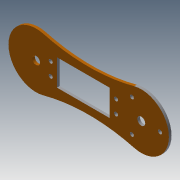
# Autodesk Inventor part: dibond_strana(b)
Saved by Autodesk Inventor 2013 (Build 170138000, 138)
## iProperties
Created: 2013-05-11
Part Number: dibond_strana(b)
Material: Generic
Document SubType Name: Modeling
Designer: idle-rug
Density: 1 g/cm^3
Author: idle-rug
Autodesk Inventor part; units mm, degrees
ref_plane "YZ Plane" through (0, 0, 0) normal (1, 0, 0) x (0, 1, 0)
ref_plane "XZ Plane" through (0, 0, 0) normal (0, 1, 0) x (-1, 0, 0)
ref_plane "XY Plane" through (0, 0, 0) normal (0, 0, 1) x (1, 0, 0)
sketch "Sketch1" plane through (0, 0, 0) normal (0, 1, 0) x (-1, 0, 0)
  line L0 (-50.5, -21) -> (-38.580998, -21)
  line L1 (-50.5, -21) -> (-38.580998, -21)
  line L2 (-50.5, 21) -> (-38.580998, 21)
  arc A0 (-50.5, 21) -> (-50.5, -21) centre (-50.5, 0) ccw
  circle A1 centre (40, 0) radius 3
  line L3 (-71.5, 0) -> (-61.5, 0)
  line L4 (-50.5, 21) -> (-37.146287, 21)
  arc A2 (-37.146287, 21) -> (34.589084, 20.290934) centre (0, 150) ccw
  line L5 (-50.5, -21) -> (-37.146287, -21)
  arc A3 (34.589084, -20.290934) -> (-37.146287, -21) centre (0, -150) ccw
  circle A4 centre (-61.5, 0) radius 2
  line L6 (40, 0) -> (20, 0)
  circle A5 centre (20, 0) radius 2
  arc A6 (37.224562, -20.815786) -> (37.224562, 20.815786) centre (40, 0) ccw
  arc A7 (34.589084, -20.290934) -> (34.589084, 20.290934) centre (40, 0) ccw
  point P0 (0, 0)
  point P1 (0, 0)
  dimension "d1" = 6
  dimension "d3" = 10
  dimension "d5" = 4
  dimension "d7" = 4
  constraints: 14 end point, 11 point on circle, 8 centre point, 5 tangent, 2 coincident, 1 point on line
  measures "d1" diameter of A1
  measures "d3" distance of L3.start L3.end
  measures "d5" diameter of A4
  measures "d7" diameter of A5
extrude "Extrusion1" add sketch "Sketch1" along normal blind 2
sketch "Sketch2" plane through (0, 2, 0) normal (0, 1, 0) x (1, 0, 0)
  circle A0 centre (-54.25, 0) radius 1.5
  circle A1 centre (-32.875, 12.340862) radius 1.5
  circle A2 centre (-32.875, -12.340862) radius 1.5
  point P0 (0, 0)
  dimension "d11" = 3
  dimension "d14" = 3
  dimension "d15" = 3
  constraints: 3 centre point
  measures "d11" diameter of A0
  measures "d14" diameter of A1
  measures "d15" diameter of A2
extrude "Extrusion2" cut sketch "Sketch2" against normal blind 2
sketch "Sketch3" plane through (0, 2, 0) normal (0, 1, 0) x (1, 0, 0)
  line L0 (37.146287, -21) -> (50.5, -21)
  arc A0 (50.5, -21) -> (50.5, 21) centre (50.5, 0) ccw
  line L1 (50.5, 0) -> (40, 0)
  circle A1 centre (40, 0) radius 3
  point P0 (0, 0)
  dimension "d18" = 10.5
  dimension "d19" = 6
  constraints: 2 end point, 1 centre point, 1 coincident, 1 parallel
  measures "d18" distance of L1.start L1.end
  measures "d19" diameter of A1
extrude "Extrusion3" cut sketch "Sketch3" against normal blind 2
sketch "Sketch4" plane through (0, 0, 0) normal (0, -1, 0) x (1, 0, 0)
  circle A0 centre (40, 0) radius 3
  line L0 (40, 0) -> (54.25, 0) construction
  line L1 (40, 0) -> (54.25, 0) construction
  line L2 (40, 0) -> (54.25, 0) construction
  line L3 (40, 0) -> (54.25, 0) construction
  circle A1 centre (47.125, 12.340862) radius 1.5
  circle A2 centre (25.75, 0) radius 1.5
  circle A3 centre (47.125, -12.340862) radius 1.5
  point P0 (0, 0)
  dimension "d33" = 3
  dimension "d34" = 3
  dimension "d35" = 3
  constraints: 8 end point, 4 horizontal, 3 centre point, 1 coincident
  measures "d33" diameter of A1
  measures "d34" diameter of A2
  measures "d35" diameter of A3
extrude "Extrusion4" cut sketch "Sketch4" against normal blind 2 contours A1 | A2 | A3
sketch "Sketch5" plane through (0, 0, 0) normal (0, -1, 0) x (1, 0, 0)
  line L0 (50.5, -21) -> (37.146287, -21)
  arc A0 (50.5, -21) -> (50.5, 21) centre (50.5, 0) ccw
  line L1 (37.146287, 21) -> (50.5, 21)
  arc A1 (-34.589084, 20.290934) -> (37.146287, 21) centre (0, 150) ccw
  arc A2 (-34.589084, 20.290934) -> (-34.589084, -20.290934) centre (-40, 0) ccw
  arc A3 (37.146287, -21) -> (-34.589084, -20.290934) centre (0, -150) ccw
  line L2 (74.65, 0) -> (104.15, 0)
  line L3 (74.65, 0) -> (63.95, 0)
  line L4 (37.146287, 21) -> (104.15, 21)
  line L5 (104.15, 21) -> (37.146287, 21)
  line L6 (37.146287, -21) -> (104.15, -21)
  line L7 (63.95, 0) -> (104.15, 0)
  line L8 (104.15, 10) -> (63.95, 10)
  line L9 (63.95, 10) -> (63.95, -10)
  line L10 (63.95, -10) -> (104.15, -10)
  line L11 (104.15, -10) -> (104.15, 10)
  line L12 (104.15, 10) -> (63.95, -10) construction
  line L13 (63.95, 10) -> (104.15, -10) construction
  line L14 (104.15, -4.95) -> (104.15, -10)
  line L15 (104.15, 4.95) -> (104.15, 10)
  arc A4 (104.15, -21) -> (104.15, 21) centre (104.15, 0) ccw
  circle A5 centre (108.9, 4.95) radius 1.5
  circle A6 centre (108.9, -4.95) radius 1.5
  circle A7 centre (59.2, 4.95) radius 1.5
  circle A8 centre (59.2, -4.95) radius 1.5
  point P0 (0, 0)
  point P1 (84.05, 0)
  dimension "d46" = 29.5
  dimension "d48" = 10.7
  dimension "d49" = 40.2
  dimension "d57" = 3
  dimension "d58" = 3
  constraints: 28 end point, 5 centre point, 5 parallel, 3 midpoint, 2 collinear, 2 horizontal, 2 point on circle, 2 tangent, 1 perpendicular
  measures "d46" distance of L2.start L2.end
  measures "d48" distance of L2.start L3.end
  measures "d49" distance of L10.end L9.end
  measures "d57" diameter of A5
  measures "d58" diameter of A6
extrude "Extrusion5" add sketch "Sketch5" against normal blind 2 contours A0 L10 L11 L8 L4 A4 L6
sketch "Sketch6" plane through (0, 0, 0) normal (0, -1, 0) x (1, 0, 0)
  arc A0 (68.966185, -10) -> (68.966185, 10) centre (50.5, 0) ccw
  line L0 (68.966185, 10) -> (104.15, 10)
  line L1 (104.15, 10) -> (104.15, -10)
  line L2 (104.15, -10) -> (68.966185, -10)
  line L3 (104.15, 10) -> (63.95, 10)
  line L4 (63.95, 10) -> (63.95, -10)
  line L5 (63.95, -10) -> (104.15, -10)
  line L6 (104.15, -10) -> (104.15, 10)
  point P0 (0, 0)
  dimension "d65" = 40.2
  dimension "d66" = 20
  constraints: 8 end point, 1 collinear, 1 perpendicular, 1 point on line
  measures "d65" distance of L0.end L3.end
  measures "d66" distance of L3.end L4.end
extrude "Extrusion6" cut sketch "Sketch6" against normal blind 2 contours L5 L4 L3 A0
sketch "Sketch7" plane through (0, 0, 0) normal (0, -1, 0) x (1, 0, 0)
  circle A0 centre (61.5, 0) radius 2 projected
  point P0 (0, 0)
extrude "Extrusion7" add sketch "Sketch7" against normal blind 2
sketch "Sketch8" plane through (0, 0, 0) normal (0, -1, 0) x (1, 0, 0)
  circle A0 centre (108.9, 4.95) radius 1.5 projected
  circle A1 centre (108.9, -4.95) radius 1.5 projected
  line L0 (104.15, 10) -> (104.15, -10) projected
  line L1 (108.9, 4.95) -> (59.2, 4.95)
  line L2 (108.9, -4.95) -> (59.2, -4.95)
  circle A2 centre (59.2, 4.95) radius 1.5
  circle A3 centre (59.2, -4.95) radius 1.5
  point P0 (0, 0)
  dimension "d71" = 49.7
  dimension "d72" = 49.7
  dimension "d73" = 3
  dimension "d74" = 3
  constraints: 4 end point, 2 centre point, 2 coincident, 1 parallel, 1 perpendicular
  measures "d71" distance of L1.start L1.end
  measures "d72" distance of L2.start L2.end
  measures "d73" diameter of A2
  measures "d74" diameter of A3
extrude "Extrusion8" cut sketch "Sketch8" against normal blind 2 contours A2 | A3
sketch "Sketch9" plane through (0, 0, 0) normal (0, -1, 0) x (1, 0, 0)
  arc A0 (-34.589084, 20.290934) -> (37.146287, 21) centre (0, 150) ccw
  circle A1 centre (40, 0) radius 3
  circle A2 centre (47.125, -12.340862) radius 1.5
  circle A3 centre (47.125, 12.340862) radius 1.5
  circle A4 centre (25.75, 0) radius 1.5
  circle A5 centre (40, 0) radius 21
  point P0 (0, 0)
  constraints: 1 centre point, 1 coincident, 1 tangent
extrude "Extrusion9" add sketch "Sketch9" along normal blind 2
sketch "Sketch10" plane through (0, 0, 0) normal (0, -1, 0) x (1, 0, 0)
  arc A0 (60.07327, 6.16959) -> (40, 21) centre (40, 0) ccw
  arc A1 (60.554075, 4.304647) -> (60.07327, 6.16959) centre (59.2, 4.95) ccw
  arc A2 (60.554075, -4.304647) -> (60.554075, 4.304647) centre (40, 0) ccw
  arc A3 (60.07327, -6.16959) -> (60.554075, -4.304647) centre (59.2, -4.95) ccw
  arc A4 (40, -21) -> (60.07327, -6.16959) centre (40, 0) ccw
  line L0 (104.15, -21) -> (40, -21)
  arc A5 (104.15, -21) -> (104.15, 21) centre (104.15, 0) ccw
  line L1 (40, 21) -> (104.15, 21)
  circle A6 centre (108.9, 4.95) radius 1.5
  circle A7 centre (108.9, -4.95) radius 1.5
  line L2 (104.15, -10) -> (63.95, -10)
  line L3 (63.95, -10) -> (63.95, 10)
  line L4 (63.95, 10) -> (104.15, 10)
  line L5 (104.15, 10) -> (104.15, -10)
  point P0 (0, 0)
extrude "Extrusion10" cut sketch "Sketch10" against normal blind 2
sketch "Sketch11" plane through (40, -2, 0) normal (0, -1, 0) x (1, 0, 0)
  circle A0 centre (0, 0) radius 3
  circle A1 centre (-14.25, 0) radius 1.5
  circle A2 centre (7.125, 12.340862) radius 1.5
  circle A3 centre (7.125, -12.340862) radius 1.5
  circle A4 centre (0, 0) radius 21
  point P0 (-40, 0)
extrude "Extrusion11" cut sketch "Sketch11" against normal blind 2
sketch "Sketch12" plane through (0, 0, 0) normal (0, -1, 0) x (1, 0, 0)
  arc A0 (60.554075, -4.304647) -> (60.07327, -6.16959) centre (59.2, -4.95) ccw
  arc A1 (60.07327, 6.16959) -> (60.554075, 4.304647) centre (59.2, 4.95) ccw
  circle A2 centre (59.2, -4.95) radius 1.5
  circle A3 centre (59.2, 4.95) radius 1.5
  point P0 (0, 0)
  constraints: 2 coincident, 1 centre point, 1 concentric, 3 other
extrude "Extrusion12" add sketch "Sketch12" against normal blind 2
sketch "Sketch13" plane through (0, 0, 0) normal (0, -1, 0) x (1, 0, 0)
  circle A0 centre (25.75, 0) radius 1.5
  circle A1 centre (47.125, 12.340862) radius 1.5
  circle A2 centre (47.125, -12.340862) radius 1.5
  circle A3 centre (40, 0) radius 3
  arc A4 (37.146287, -21) -> (-34.589084, -20.290934) centre (0, -150) ccw
  arc A5 (60.07327, 6.16959) -> (40, 21) centre (40, 0) ccw
  circle A6 centre (40, 0) radius 21
  point P0 (0, 0)
  constraints: 1 centre point, 1 coincident, 1 tangent
extrude "Extrusion13" cut sketch "Sketch13" against normal blind 2
sketch "Sketch14" plane through (0, 0, 0) normal (0, -1, 0) x (1, 0, 0)
  arc A0 (60.07327, -6.16959) -> (60.554075, -4.304647) centre (40, 0) ccw
  arc A1 (60.07327, -6.16959) -> (60.554075, -4.304647) centre (59.2, -4.95) ccw
  point P0 (0, 0)
sketch "Sketch15" plane through (0, 0, 0) normal (0, -1, 0) x (1, 0, 0)
  arc A0 (60.554075, 4.304647) -> (60.07327, 6.16959) centre (40, 0) ccw
  arc A1 (60.554075, 4.304647) -> (60.07327, 6.16959) centre (59.2, 4.95) ccw
  point P0 (0, 0)
sketch "Sketch16" plane through (0, 0, 0) normal (0, -1, 0) x (1, 0, 0)
  arc A0 (40, 21) -> (34.589084, 20.290934) centre (40, 0) ccw
  line L0 (37.146287, 21) -> (40, 21)
  arc A1 (34.589084, 20.290934) -> (37.146287, 21) centre (0, 150) ccw
  point P0 (0, 0)
sketch "Sketch17" plane through (0, 0, 0) normal (0, -1, 0) x (1, 0, 0)
  arc A0 (34.589084, -20.290934) -> (40, -21) centre (40, 0) ccw
  arc A1 (37.146287, -21) -> (34.589084, -20.290934) centre (0, -150) ccw
  line L0 (40, -21) -> (37.146287, -21)
  point P0 (0, 0)
extrude "Extrusion14" cut sketch "Sketch17" against normal blind 2
extrude "Extrusion15" cut sketch "Sketch14" against normal blind 2
extrude "Extrusion16" cut sketch "Sketch15" against normal blind 2
extrude "Extrusion17" cut sketch "Sketch16" against normal blind 2
sketch "Sketch18" plane through (0, 0, 0) normal (0, -1, 0) x (1, 0, 0)
  arc A0 (34.589084, 20.290934) -> (34.589084, -20.290934) centre (40, 0) ccw
  circle A1 centre (40, 0) radius 21
  circle A2 centre (40, 0) radius 3
  point P0 (0, 0)
  dimension "d95" = 6
  constraints: 2 centre point, 2 coincident, 1 concentric
  measures "d95" diameter of A2
extrude "Extrusion18" add sketch "Sketch18" against normal blind 2
sketch "Sketch19" plane through (0, 2, 0) normal (0, 1, 0) x (1, 0, 0)
  arc A0 (34.589084, -20.290934) -> (34.589084, 20.290934) centre (40, 0) ccw
  circle A1 centre (40, 0) radius 17.325
  circle A2 centre (5.35, 0) radius 17.325
  line L0 (16.05, 10) -> (-24.15, 10)
  line L1 (-24.15, 10) -> (-24.15, -10)
  line L2 (-24.15, -10) -> (16.05, -10)
  line L3 (16.05, -10) -> (16.05, 10)
  line L4 (16.05, 10) -> (-24.15, -10) construction
  line L5 (-24.15, 10) -> (16.05, -10) construction
  line L6 (16.05, -4.95) -> (16.05, -10)
  line L7 (16.05, 4.95) -> (16.05, 10)
  circle A3 centre (20.8, 4.95) radius 1.5
  circle A4 centre (20.8, -4.95) radius 1.5
  line L8 (20.8, 4.95) -> (-28.9, 4.95)
  line L9 (20.8, -4.95) -> (-28.9, -4.95)
  circle A5 centre (-28.9, 4.95) radius 1.5
  circle A6 centre (-28.9, -4.95) radius 1.5
  point P0 (0, 0)
  point P1 (-4.05, 0)
  dimension "d100" = 34.65
  dimension "d103" = 40.2
  dimension "d104" = 20
  dimension "d109" = 3
  dimension "d110" = 3
  dimension "d111" = 49.7
  dimension "d112" = 49.7
  dimension "d113" = 3
  dimension "d114" = 3
  constraints: 20 end point, 6 centre point, 3 coincident, 3 parallel, 2 midpoint, 2 perpendicular, 1 horizontal
  measures "d100" diameter of A2
  measures "d103" distance of L2.end L1.end
  measures "d104" distance of L1.end L0.end
  measures "d109" diameter of A3
  measures "d110" diameter of A4
  measures "d111" distance of L8.start L8.end
  measures "d112" distance of L9.start L9.end
  measures "d113" diameter of A5
  measures "d114" diameter of A6
extrude "Extrusion19" cut sketch "Sketch19" against normal blind 2 contours A3 A2 | A2 A3 | A4 A2 | A2 A4 | L0 L3 L8 A2 | A2 L8 L1 L0 | L3 L9 A2 L8 | L2 L1 L9 A2 | A2 L9 L3 L2 | A2 L9 L1 L8 | A5 | A6
sketch "Sketch20" plane through (0, 0, 0) normal (0, -1, 0) x (1, 0, 0)
  arc A0 (34.589084, -20.290934) -> (34.589084, 20.290934) centre (40, 0) ccw
  line L0 (40, 0) -> (54.25, 0) construction
  line L1 (40, 0) -> (54.25, 0) construction
  circle A1 centre (32.875, 12.340862) radius 1.5
  circle A2 centre (32.875, -12.340862) radius 1.5
  circle A3 centre (54.25, 0) radius 1.5
  point P0 (0, 0)
  dimension "d120" = 3
  dimension "d121" = 3
  constraints: 4 end point, 3 centre point, 2 coincident, 2 horizontal
  measures "d120" diameter of A1
  measures "d121" diameter of A2
extrude "Extrusion20" cut sketch "Sketch20" against normal blind 2
sketch "Sketch21" plane through (0, 0, 0) normal (0, -1, 0) x (1, 0, 0)
  circle A0 centre (-32.875, -12.340862) radius 1.5
  circle A1 centre (-54.25, 0) radius 1.5
  circle A2 centre (-32.875, 12.340862) radius 1.5
  point P0 (0, 0)
extrude "Extrusion21" add sketch "Sketch21" against normal blind 2
body "Solid1"
